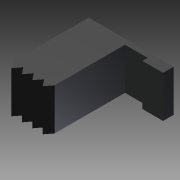
# Autodesk Inventor part: AS11CHcright
Saved by Autodesk Inventor 2011 SP1 (Build 150282100, 282)
## iProperties
Created: 2018-06-01
Part Number: AS11CHcright
Catalog Web Link: www.cadenas.de
Description: AS - Series - Actuators C for Right Angle-
Vendor: NKKSWITCHES
Document SubType Name: Modeling
Designer: psAdmin
Manufacturer: NKKSWITCHES
Mass: 0.0285264 g
Surface Area: 0.72923 cm^2
Volume: 0.0285264 cm^3
Density: 1 g/cm^3
Category: PARTsolutions
Company: NKKSWITCHES
Title: AS11CHcright
Author: Cadenas PARTsolutions
PSOL_IDENT_0: {$CADENAS_DATA\23d-libs\nkkswitches\slides\as\parts\as_actu_c_right.prj},222 {VTYP=3D},{NB=AS11CHcri
PSOL_IDENT_1: ght},{LINA=AS11CHcright},{NN=AS - Series - Actuators C for Right Angle},{DATE=11.10.2017 10:53:50},{
PSOL_IDENT_2: GEOMDATE=09.12.2008 09:29:00},{VERSION=},{LINEID=10},{LINESUBID=-1},{WBVAR=PLS,CRCTS,ACTU,TRMNLS}  {
PSOL_IDENT_3: NB=AS11CHcright},{LINA=AS11CHcright},{KT=DUMMY},{PN=AS11CH},{SRS=AS},{PLS=1},{CRCTS=1},{CRCTSALG=  '
PSOL_IDENT_4: 1', '1 - ON/NONE/OFF','2', '2 - ON/NONE/ON', '3', '3 - ON/OFF/ON' },{ACTU=C},{TRMNLS=H},{CCLR=0.50,0
PSOL_IDENT_5: .50,0.50,0.00}
NN: AS - Series - Actuators C for Right Angle
NB: AS11CHcright
NBSYN: $PN.cright
LINA: AS11CHcright
PN: AS11CH
SRS: AS
PLS: 1 - SPST/SPDT
CRCTS: 1 - ON/NONE/OFF
ACTU: C - .150"(3,8mm)Long
TRMNLS: H - Right Angle with Bracket
SUPPLIER: NKKSWITCHES
ARTICLENO: AS11CHcright
BOMINFO: AS11CHcright
CREATOR: CADENAS GmbH
Autodesk Inventor part; units mm, degrees
sketch "Sketch_1" plane through (0, 0, 0) normal (0, 1, 0) x (-1, 0, 0)
  line L0 (0, 3.7338) -> (-0.2984, 4.1148)
  line L1 (-0.2984, 4.1148) -> (-0.5969, 3.7338)
  line L2 (-0.5969, 3.7338) -> (-0.8954, 4.1148)
  line L3 (-0.8954, 4.1148) -> (-1.1938, 3.7338)
  line L4 (-1.1938, 3.7338) -> (-1.4884, 4.1148)
  line L5 (-1.4884, 4.1148) -> (-1.7869, 3.7338)
  line L6 (-1.7869, 3.7338) -> (-2.0853, 4.1148)
  line L7 (-2.0853, 4.1148) -> (-2.3876, 3.7338)
  line L8 (-2.3876, 3.7338) -> (-2.3876, 0)
  line L9 (-2.3876, 0) -> (0, 0)
  line L10 (0, 0) -> (0, 3.7338)
  constraints: 22 end point
extrude "Extrusion1" add sketch "Sketch_1" along normal blind 2.3876
sketch "Sketch_2" plane through (0, 0, 0) normal (0, 0, 1) x (1, 0, 0)
  line L0 (0, 2.3876) -> (0, 0)
  line L1 (0, 0) -> (4.8768, 0)
  line L2 (4.8768, 0) -> (4.8768, 2.3876)
  line L3 (4.8768, 2.3876) -> (0, 2.3876)
  constraints: 8 end point
extrude "Extrusion2" add sketch "Sketch_2" against normal blind 0.6096
sketch "Sketch_3" plane through (0, 0, 0) normal (0, 0, 1) x (1, 0, 0)
  line L0 (2.3876, 2.3876) -> (2.3876, 0)
  line L1 (2.3876, 0) -> (3.683, 0)
  line L2 (3.683, 0) -> (3.683, 2.3876)
  line L3 (3.683, 2.3876) -> (2.3876, 2.3876)
  constraints: 8 end point
extrude "Extrusion3" cut sketch "Sketch_3" against normal blind 0.3048
ref_plane "body_right1c_XY" through (2.3876, 1.1938, -0.6096) normal (0, 0, 1) x (1, 0, 0)
ref_plane "body_right1c_YZ" through (2.3876, 1.1938, -0.6096) normal (1, 0, 0) x (0, 1, 0)
ref_plane "body_right1c_ZX" through (2.3876, 1.1938, -0.6096) normal (0, 1, 0) x (0, 0, 1)
body "Solid1"
